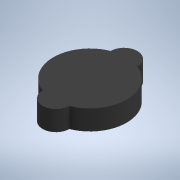
# Autodesk Inventor part: buttons_battery
Saved by Autodesk Inventor 2020 (Build 240168000, 168)
## iProperties
Created: 2019-11-16
Part Number: buttons_battery
Material: Generic
Document SubType Name: Modeling
Designer: suchanek
Density: 1 g/cm^3
Appearance: Default
Author: suchanek
Autodesk Inventor part; units mm, degrees
ref_plane "YZ Plane" through (0, 0, 0) normal (1, 0, 0) x (0, 1, 0)
ref_plane "XZ Plane" through (0, 0, 0) normal (0, 1, 0) x (-1, 0, 0)
ref_plane "XY Plane" through (0, 0, 0) normal (0, 0, 1) x (1, 0, 0)
sketch "Sketch1" plane through (0, 0, 0) normal (0, 1, 0) x (-1, 0, 0)
  circle A0 centre (0, 0) radius 11
  arc A1 (4, 10.247) -> (-4, 10.247) centre (0, 10.247) ccw
  arc A2 (-4, -10.247) -> (4, -10.247) centre (0, -10.247) ccw
  dimension "d0" = 22
  dimension "d1" = 4
  constraints: 8 point on circle, 3 centre point, 2 horizontal alignment, 2 vertical alignment, 1 coincident, 1 equal radius
  measures "d0" diameter of A0
  measures "d1" radius of A1
extrude "Extrusion1" add sketch "Sketch1" along normal blind 6
body "Solid1"
